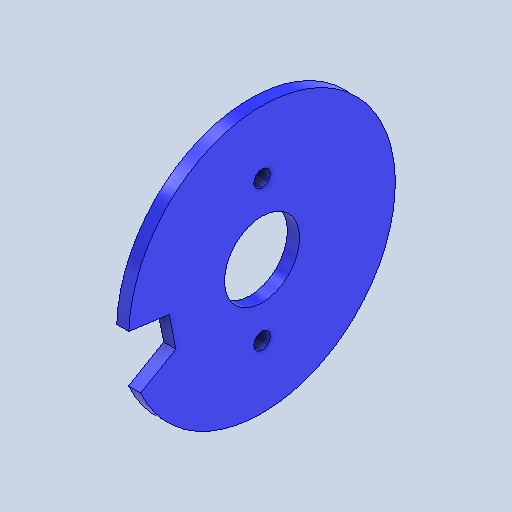
# Autodesk Inventor part: belt_liner_v1_3DP_P_F-2
Saved by Autodesk Inventor 2025.2 (Build 292293000, 293)
## iProperties
Created: 2024-12-16
Part Number: belt_liner_v1_3DP_P_F-2
Material: ABS プラスチック
Document SubType Name: Modeling
Designer: haruy
Density: 1.06 g/cm^3
Appearance: 青 - 壁塗料 - 光沢
Author: haruy
Autodesk Inventor part; units mm, degrees
ref_plane "YZ Plane" through (0, 0, 0) normal (1, 0, 0) x (0, 1, 0)
ref_plane "XZ Plane" through (0, 0, 0) normal (0, 1, 0) x (-1, 0, 0)
ref_plane "XY Plane" through (0, 0, 0) normal (0, 0, 1) x (1, 0, 0)
sketch "スケッチ3" plane through (0, 0, 0) normal (1, 0, 0) x (0, 1, 0)
  circle A0 centre (20.2536, 6.0194) radius 1.7
  circle A1 centre (-8.7464, 6.0194) radius 1.7
  line L0 (-1.3547, 23.8145) -> (-5.5771, 31.0767)
  arc A2 (-5.5771, 31.0767) -> (6.6327, 33.5054) centre (5.7536, 6.0194) ccw
  line L1 (6.6327, 33.5054) -> (5.5108, 25.1801)
  line L2 (5.5108, 25.1801) -> (-1.3547, 23.8145)
  circle A3 centre (5.7536, 6.0194) radius 7.75
  point P0 (0, 0)
  constraints: 6 end point, 4 centre point, 2 point on circle
extrude "押し出し3" add sketch "スケッチ3" along normal blind 2.5
